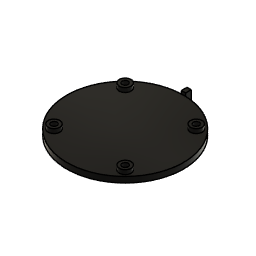
Cover V2 - USB C v5 (Autodesk Fusion 360 design; units mm, degrees)
Autodesk Fusion 360 part; units mm, degrees
sketch "Schizzo1" plane through (0, 0, 0) normal (0, 1, 0) x (1, 0, 0)
  circle A0 centre (0, 0) radius 41
  dimension "d1" = 82
  constraint coincident A0.centre origin
  measures "d1" diameter of A0
extrude "Estrusione1" add sketch "Schizzo1" along normal blind 4 makes body 1
sketch "Schizzo2" plane through (0, 4, 0) normal (0, 1, 0) x (-1, 0, 0)
  circle A0 centre (0, 0) radius 41
  line L0 (0, 0) -> (25, 0) construction
  line L1 (25, 0) -> (25, -25) construction
  circle A1 centre (25, -25) radius 2.1
  circle A2 centre (25, -25) radius 4.1
  dimension "d4" = 25
  dimension "d5" = 25
  dimension "d6" = 4.2
  dimension "d7" = 2
  constraint coincident A0.centre L0.start
  constraint horizontal L0
  constraint perpendicular L0 L1
  constraint coincident L1.end A1.centre
  measures "d4" distance of A0.centre L0.end
  measures "d5" distance of L0.end L1.end
  measures "d6" diameter of A1
extrude "Estrusione2" add sketch "Schizzo2" along normal blind 3 separate body contours A2 makes body 2
pattern_linear "Serie R2" count 2 spacing 50 along (0, 0, 1) count 2 spacing 50 along (1, 0, 0) of bodies 2 makes body 3 at (-29.0949, 6, 24.7956) makes body 4 at (20.9051, 6, -25.2044) makes body 5 at (20.9051, 6, 24.7956)
sketch "Schizzo4" plane through (0, 4, 0) normal (0, 1, 0) x (-1, 0, 0)
  circle A0 centre (0, 0) radius 41
  circle A1 centre (0, 0) radius 45
  line L0 (0, 0) -> (0, -45) construction
  line L1 (0, -40) -> (-1.5, -40)
  line L2 (0, -40) -> (1.5, -40)
  line L3 (-1.5, -40) -> (-1.5, -44.975)
  line L4 (1.5, -40) -> (1.5, -44.975)
  dimension "d23" = 90
  dimension "d24" = 1.5
  dimension "d25" = 1.5
  constraint coincident A0.centre A1.centre
  constraint coincident A1 L0.end
  constraint vertical L0
  constraint coincident L0 L1.start
  constraint perpendicular L0 L1
  constraint perpendicular L0 L2
  constraint coincident A1 L3.end
  constraint perpendicular L1 L3
  constraint coincident A1 L4.end
  constraint perpendicular L2 L4
  measures "d23" diameter of A1
  measures "d24" distance of L1.start L1.end
  measures "d25" distance of L1.start L2.end
extrude "Estrusione4" add sketch "Schizzo4" along normal blind -4 and the other way blind -2.04 contours A0 A1 L3 L4 picked at (1.1667, -42.3148) bodies 1
